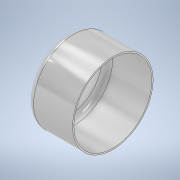
# Autodesk Inventor part: Кожух
Saved by Autodesk Inventor 2022 (Build 260153000, 153)
## iProperties
Created: 2024-04-28
Part Number: Кожух
Material: Типовые
Document SubType Name: Modeling
Designer: Pavel
Density: 1 g/cm^3
Appearance: По умолчанию
Mass: 1.0673 g
Surface Area: 43.2154 cm^2
Volume: 1.0673 cm^3
Author: Pavel
Autodesk Inventor part; units mm, degrees
ref_plane "YZ Plane" through (0, 0, 0) normal (1, 0, 0) x (0, 1, 0)
ref_plane "XZ Plane" through (0, 0, 0) normal (0, 1, 0) x (-1, 0, 0)
ref_plane "XY Plane" through (0, 0, 0) normal (0, 0, 1) x (1, 0, 0)
sketch "Эскиз1" plane through (0, 0, 0) normal (0, 1, 0) x (-1, 0, 0)
  line L0 (0, 0) -> (0, 15) construction
  line L1 (0, 15) -> (14.5, 15)
  line L2 (17, 12.5) -> (17, 1.75)
  line L3 (17, 1.75) -> (16.5, 1.75)
  line L4 (16.5, 1.75) -> (16.5, 12.5)
  line L5 (14.5, 14.5) -> (0, 14.5)
  line L6 (0, 14.5) -> (0, 15)
  arc A0 (16.5, 12.5) -> (14.5, 14.5) centre (14.5, 12.5) ccw
  arc A1 (17, 12.5) -> (14.5, 15) centre (14.5, 12.5) ccw
  line L7 (21.0213, 0) -> (-3.5036, 0) projected
  point P0 (17, 15)
  point P1 (16.5, 14.5)
  dimension "d0" = 15
  dimension "d1" = 17
  dimension "d2" = 13.25
  dimension "d3" = 0.5
  dimension "d4" = 12.75
  dimension "d5" = 2
  dimension "d6" = 2.5
  constraints: 14 end point, 5 point on line, 4 perpendicular, 4 point on circle, 4 tangent, 3 vertical, 2 centre point
  measures "d0" distance of L0.start L0.end
  measures "d1" distance of L0.end point (17, 15)
  measures "d2" distance of point (17, 15) L2.end
  measures "d3" distance of L2.end L3.end
  measures "d4" distance of L3.end point (16.5, 14.5)
  measures "d5" radius of A0
  measures "d6" radius of A1
revolve "Вращение1" add sketch "Эскиз1" angle 360 about axis through (-10, 0, 0) along (1, 0, 0)
